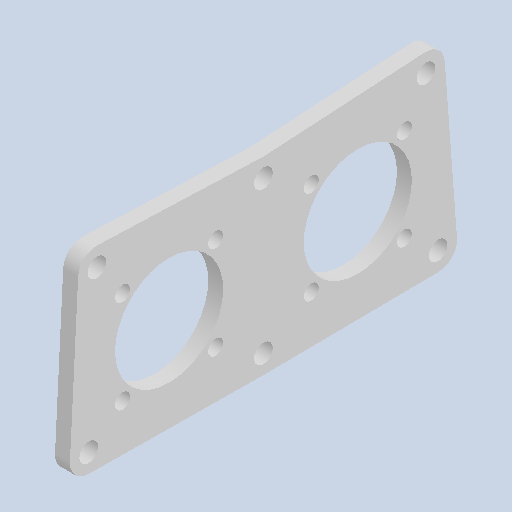
# Autodesk Inventor part: ChassiMotorMount3.0
Saved by Autodesk Inventor 2023 (Build 270158000, 158)
## iProperties
Created: 2022-09-16
Part Number: ChassiMotorMount3.0
Material: Generic
Document SubType Name: Modeling
Designer: deli
Density: 1 g/cm^3
Appearance: Default
Author: deli
Autodesk Inventor part; units mm, degrees
ref_plane "YZ Plane" through (0, 0, 0) normal (1, 0, 0) x (0, 1, 0)
ref_plane "XZ Plane" through (0, 0, 0) normal (0, 1, 0) x (-1, 0, 0)
ref_plane "XY Plane" through (0, 0, 0) normal (0, 0, 1) x (1, 0, 0)
sketch "Sketch1" plane through (0, 0, 0) normal (1, 0, 0) x (0, 1, 0)
  circle A0 centre (56.6472, 26.169) radius 2
  circle A1 centre (23.4453, 27.9096) radius 2
  circle A2 centre (39.1953, 10.8069) radius 7 construction
  circle A3 centre (23.0614, -9.2619) radius 2
  circle A4 centre (23.4453, -46.4334) radius 2
  circle A5 centre (57.3644, -43.8376) radius 2
  circle A6 centre (39.1953, -29.3308) radius 7 construction
  arc A7 (60.6445, 26.0197) -> (56.8567, 30.1635) centre (56.6472, 26.169) ccw
  circle A8 centre (55.3292, -9.2619) radius 4 construction
  arc A9 (57.6696, -47.8259) -> (61.3574, -43.6009) centre (57.3644, -43.8376) ccw
  arc A10 (19.4455, -46.4747) -> (23.7505, -50.4217) centre (23.4453, -46.4334) ccw
  arc A11 (19.0616, -9.3032) -> (19.0616, -9.3032) centre (23.0614, -9.2619) ccw
  arc A12 (23.6547, 31.9041) -> (19.4455, 27.9508) centre (23.4453, 27.9096) ccw
  line L0 (19.4455, 27.9508) -> (19.0616, -9.3032)
  line L1 (19.0616, -9.3032) -> (19.4455, -46.4747)
  line L2 (56.8567, 30.1635) -> (23.6547, 31.9041)
  line L3 (57.6696, -47.8259) -> (23.7505, -50.4217)
  arc A13 (59.332, -9.1126) -> (59.3362, -9.4986) centre (63.3292, -9.2619) ccw
  line L4 (60.6445, 26.0197) -> (59.332, -9.1126)
  line L5 (61.3574, -43.6009) -> (59.3362, -9.4986)
  line L6 (23.0614, -9.2619) -> (63.3292, -9.2619) construction
  circle A14 centre (39.1953, 10.8069) radius 11.5
  circle A15 centre (39.1953, -29.3308) radius 11.5
  circle A16 centre (49.0948, 20.7064) radius 1.6
  circle A17 centre (49.0948, 0.9074) radius 1.6
  circle A18 centre (29.2958, 0.9074) radius 1.6
  circle A19 centre (29.2958, 20.7064) radius 1.6
  circle A20 centre (29.2958, -19.4313) radius 1.6
  circle A21 centre (49.0948, -19.4313) radius 1.6
  circle A22 centre (49.0948, -39.2303) radius 1.6
  circle A23 centre (29.2958, -39.2303) radius 1.6
  line L7 (49.0948, 20.7064) -> (49.0948, 0.9074) construction
  line L8 (49.0948, 0.9074) -> (29.2958, 0.9074) construction
  line L9 (29.2958, 0.9074) -> (29.2958, 20.7064) construction
  line L10 (29.2958, 20.7064) -> (49.0948, 20.7064) construction
  line L11 (49.0948, 20.7064) -> (29.2958, 0.9074) construction
  line L12 (29.2958, 20.7064) -> (49.0948, 0.9074) construction
  line L13 (49.0948, -19.4313) -> (49.0948, -39.2303) construction
  line L14 (49.0948, -39.2303) -> (29.2958, -39.2303) construction
  line L15 (29.2958, -39.2303) -> (29.2958, -19.4313) construction
  line L16 (29.2958, -19.4313) -> (49.0948, -19.4313) construction
  line L17 (29.2958, -39.2303) -> (49.0948, -19.4313) construction
  line L18 (29.2958, -19.4313) -> (49.0948, -39.2303) construction
  circle A24 centre (56.6472, 26.169) radius 2 projected
  circle A25 centre (23.4453, 27.9096) radius 2 projected
  circle A26 centre (23.0614, -9.2619) radius 2 projected
  circle A27 centre (55.3292, -9.2619) radius 2 projected
  circle A28 centre (57.3644, -43.8376) radius 2 projected
  circle A29 centre (23.4453, -46.4334) radius 2 projected
  circle A30 centre (39.1953, 10.8069) radius 7 construction
  circle A31 centre (39.1953, -29.3308) radius 7 construction
  point P0 (0, 0)
  point P1 (67.3062, -9.2966)
  point P2 (49.3122, -19.5779)
  point P3 (21.0827, -58.3908)
  point P4 (39.1953, 10.8069)
  point P5 (39.1953, -29.3308)
  point P6 (19.3835, -56.016)
  point P7 (17.555, -42.4349)
  point P8 (17.3497, -15.1829)
  point P9 (53.615, -21.1734)
  point P10 (53.7299, -25.9433)
  point P11 (21.0179, -9.8497)
  point P12 (19.0255, -12.7465)
  dimension "d0" = 8
  dimension "d1" = 8
  dimension "d2" = 8
  dimension "d3" = 8
  dimension "d4" = 8
  dimension "d5" = 8
  dimension "d6" = 8
  dimension "d8" = 23
  dimension "d9" = 23
  dimension "d12" = 3.2
  dimension "d13" = 3.2
  dimension "d14" = 3.2
  dimension "d15" = 3.2
  dimension "d16" = 3.2
  dimension "d17" = 3.2
  dimension "d18" = 3.2
  dimension "d19" = 3.2
  dimension "d20" = 28
  dimension "d21" = 0
  dimension "d22" = 0
  dimension "d23" = 28
  constraints: 38 end point, 24 centre point, 12 point on circle, 12 tangent, 8 coincident, 8 concentric, 6 perpendicular, 5 equal radius, 4 midpoint, 4 vertical, 1 horizontal, 1 point on line
  measures "d0" diameter of A7
  measures "d1" diameter of A12
  measures "d2" diameter of A11
  measures "d3" diameter of A8
  measures "d4" diameter of A9
  measures "d5" diameter of A10
  measures "d6" diameter of A13
  measures "d8" diameter of A14
  measures "d9" diameter of A15
  measures "d12" diameter of A16
  measures "d13" diameter of A17
  measures "d14" diameter of A18
  measures "d15" diameter of A19
  measures "d16" diameter of A20
  measures "d17" diameter of A21
  measures "d18" diameter of A22
  measures "d19" diameter of A23
  measures "d20" distance of L7.start L8.end
  measures "d21" distance of point (39.195, 10.807) A2.centre
  measures "d22" distance of A6.centre point (39.195, -29.331)
  measures "d23" distance of L14.end L13.start
extrude "Extrusion1" add sketch "Sketch1" along normal blind 3.175 contours A11 | L4 A13 L5 A9 L3 A10 L1 L0 A12 L2 A7
equation "\"d1\" = d0"
equation "\"d2\" = d0"
equation "\"d3\" = d0"
equation "\"d4\" = d0"
equation "\"d5\" = d0"
equation "\"d6\" = d0"
equation "\"d9\" = d8"
equation "\"d13\" = d12"
equation "\"d14\" = d12"
equation "\"d15\" = d12"
equation "\"d16\" = d12"
equation "\"d17\" = d12"
equation "\"d18\" = d12"
equation "\"d19\" = d12"
equation "\"d23\" = d20"
body "Solid1"
